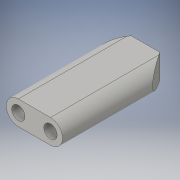
# Autodesk Inventor part: Splitter
Saved by Autodesk Inventor 2016 (Build 200138000, 138)
## iProperties
Created: 2015-07-29
Part Number: Splitter
Material: Generic
Document SubType Name: Modeling
Designer: Nancy
Density: 1 g/cm^3
Appearance: Default
Author: Nancy
Autodesk Inventor part; units mm, degrees
ref_plane "YZ Plane" through (0, 0, 0) normal (1, 0, 0) x (0, 1, 0)
ref_plane "XZ Plane" through (0, 0, 0) normal (0, 1, 0) x (-1, 0, 0)
ref_plane "XY Plane" through (0, 0, 0) normal (0, 0, 1) x (1, 0, 0)
sketch "Sketch5" plane through (0, 0, 0) normal (0, 0, 1) x (1, 0, 0)
  line L0 (-2.8956, 2.1593) -> (2.8956, 2.1593)
  arc A0 (2.8956, -2.1593) -> (2.8956, 2.1593) centre (2.8956, 0) ccw
  line L1 (2.8956, -2.1593) -> (-2.8956, -2.1593)
  arc A1 (-2.8956, 2.1593) -> (-2.8956, -2.1593) centre (-2.8956, 0) ccw
  point P0 (0, 0)
  dimension "d44" = 2.8956
  dimension "d45" = 2.8956
  constraints: 4 end point, 4 point on circle, 3 tangent, 2 centre point, 2 horizontal
  measures "d44" distance of point (0, 0) A1.centre
  measures "d45" distance of point (0, 0) A0.centre
extrude "Extrusion1" add sketch "Sketch5" along normal blind 20
sketch "Sketch6" plane through (0, 0, 20) normal (0, 0, 1) x (1, 0, 0)
  circle A0 centre (2.8956, 0) radius 1.1906
  circle A1 centre (-2.8956, 0) radius 1.1906
  point P0 (0, 0)
  dimension "d28" = 2.3813
  dimension "d29" = 2.8956
  dimension "d30" = 2.8956
  dimension "d31" = 2.3813
  constraints: 2 centre point
  measures "d28" diameter of A0
  measures "d29" distance of point (0, 0) A0.centre
  measures "d30" distance of point (0, 0) A1.centre
  measures "d31" diameter of A1
extrude "Extrusion2" cut sketch "Sketch6" against normal blind 15
sketch "Sketch7" plane through (0, 0, 0) normal (0, 0, -1) x (-1, 0, 0)
  circle A0 centre (0, 0) radius 1.1906
  dimension "d34" = 2.3813
  constraints: 1 centre point, 1 coincident
  measures "d34" diameter of A0
extrude "Extrusion3" cut sketch "Sketch7" against normal blind 15
sketch "Sketch8" plane through (-2.8956, 2.1593, 0) normal (0, 1, 0) x (1, 0, 0)
  line L0 (7.9505, 0) -> (7.9505, -20) projected
  line L1 (7.9505, -3.81) -> (5.4781, 0)
  line L2 (0, 0) -> (5.7912, 0) projected
  line L3 (0.3048, 0) -> (-2.1593, -3.81)
  line L4 (-2.1593, 0) -> (-2.1593, -20) projected
  line L5 (5.4781, 0) -> (7.9505, 0)
  line L6 (0.3048, 0) -> (-2.1593, 0)
  line L7 (5.7912, 0) -> (0, 0) projected
  point P0 (2.8956, 0)
  dimension "d37" = 2.5825
  dimension "d38" = 2.5908
  dimension "d39" = 3.81
  dimension "d40" = 3.81
  constraints: 8 end point, 4 point on line, 1 collinear, 1 horizontal
  measures "d37" distance of point (2.896, 0) L1.end
  measures "d38" distance of L3.start point (2.896, 0)
  measures "d39" vertical distance of L3.start L3.end
  measures "d40" vertical distance of L1.end L1.start
extrude "Extrusion4" cut sketch "Sketch8" against normal blind 15
body "Solid2"
